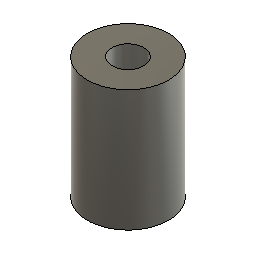
drill bit threaded holder v2 (Autodesk Fusion 360 design; units mm, degrees)
Autodesk Fusion 360 part; units mm, degrees
cylinder "CylinderPrimitive1" add diameter 10 height 15 placed x (1, 0, 0) y (0, 0, -1) z (0, 1, 0) at (0, 0, 0) makes body 1
cylinder "CylinderPrimitive2" add diameter 8 height 12 placed x (1, 0, 0) y (0, 0, -1) z (0, 1, 0) at (0, 0, 0) separate body makes body 2
combine "Combine1" operation cut target body 1 tool bodies 2
cylinder "CylinderPrimitive3" cut diameter 3.9 height 20 placed x (1, 0, 0) y (0, 0, -1) z (0, 1, 0) at (0, 0, 0) bodies 1
thread "Thread1" "ISO Metric profile 8.0 M8x0.75 6H" major diameter 8.1201 minor diameter 7.2831 pitch 0.75 angle 60 modelled right hand crest width 0.0938 on face at (3.9801, 8, 0.3983) crest through (3.6416, -0.4219, 0) on bodies 1
